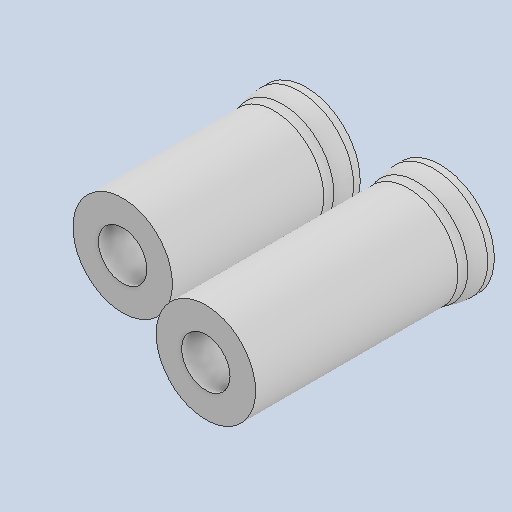
# Autodesk Inventor part: Shaft
Saved by Autodesk Inventor 2023.1 (Build 271208000, 208)
## iProperties
Created: 2022-09-21
Part Number: Shaft
Material: Generic
Document SubType Name: Modeling
Designer: Windows10
Density: 1 g/cm^3
Appearance: Default
Author: Windows10
Autodesk Inventor part; units mm, degrees
ref_plane "YZ Plane" through (0, 0, 0) normal (1, 0, 0) x (0, 1, 0)
ref_plane "XZ Plane" through (0, 0, 0) normal (0, 1, 0) x (-1, 0, 0)
ref_plane "XY Plane" through (0, 0, 0) normal (0, 0, 1) x (1, 0, 0)
sketch "Sketch1" plane through (0, 0, 0) normal (0, 0, 1) x (1, 0, 0)
  circle A0 centre (0, 0) radius 1.95
  circle A1 centre (0, 0) radius 0.95
  circle A2 centre (4.7707, 0) radius 1.95
  circle A3 centre (4.7707, 0) radius 0.95
  circle A4 centre (-5.264, 0) radius 1.95
  circle A5 centre (-5.264, 0) radius 0.95
  dimension "d0" = 3.9
  dimension "d6" = 1.9
  dimension "d9" = 3.9
  dimension "d10" = 1.9
  dimension "d13" = 3.9
  dimension "d14" = 1.9
  constraints: 6 centre point, 4 coincident
  measures "d0" diameter of A0
  measures "d6" diameter of A1
  measures "d9" diameter of A2
  measures "d10" diameter of A3
  measures "d13" diameter of A4
  measures "d14" diameter of A5
extrude "Extrusion1" add sketch "Sketch1" along normal blind 9.2 contours A0
extrude "Extrusion5" add sketch "Sketch1" along normal blind 7.2 separate body contours A4
sketch "Sketch6" plane through (-5.264, 0, 0) normal (0, 0, -1) x (-1, 0, 0)
  circle A0 centre (0, 0) radius 1.95 projected
  circle A1 centre (0, 0) radius 0.95 projected
  circle A2 centre (-5.264, 0) radius 1.95 projected
  circle A3 centre (-5.264, 0) radius 0.95 projected
  circle A4 centre (-10.0347, 0) radius 1.95 projected
  circle A5 centre (-10.0347, 0) radius 0.95 projected
  circle A6 centre (0, 0) radius 2.12
  circle A7 centre (-5.264, 0) radius 2.12
  circle A8 centre (-10.0347, 0) radius 2.15
  dimension "d19" = 0.17
  dimension "d20" = 0.17
  dimension "d21" = 0.17
  constraints: 3 centre point
  measures "d19" radial gap between concentric circles of A0 A6
  measures "d20" radial gap between concentric circles of A2 A7
extrude "Extrusion7" add sketch "Sketch6" against normal blind 0.7 contours A6 bodies 2
extrude "Extrusion8" add sketch "Sketch6" against normal blind 0.7 contours A7 bodies 1
fillet "Fillet1" radius 1 2 edges at (-1.95, 0, 0.7) (-7.214, 0, 0.7)
fillet "Fillet2" radius 2 4 edges at (0, -2.12, 0.7) (0, 2.12, 0.7) (-5.264, -2.12, 0.7) (-5.264, 2.12, 0.7)
equation "\"d6\" = d14"
equation "\"d10\" = d6"
equation "\"d20\" = d19"
equation "\"d21\" = d19"
